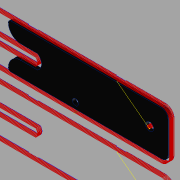
# Autodesk Inventor part: wheel_mount_brake
Saved by Autodesk Inventor 2021.3 (Build 253353000, 353)
## iProperties
Created: 2021-07-08
Part Number: wheel_mount_brake
Material: アルミニウム 6061
Document SubType Name: Modeling
Designer: gisen
Density: 2.7 g/cm^3
Appearance: アルミニウム - フラット
Author: gisen
Autodesk Inventor part; units mm, degrees
ref_plane "YZ Plane" through (0, 0, 0) normal (1, 0, 0) x (0, 1, 0)
ref_plane "XZ Plane" through (0, 0, 0) normal (0, 1, 0) x (-1, 0, 0)
ref_plane "XY Plane" through (0, 0, 0) normal (0, 0, 1) x (1, 0, 0)
ref_plane "作業平面1" through (0, 0, 0) normal (0, 0, 1) x (1, 0, 0)
sketch "スケッチ2" plane through (0, 0, 0) normal (0, 0, 1) x (1, 0, 0)
  line L0 (110, -57) -> (-20, -57)
  line L1 (-20, -57) -> (-20, -93)
  line L2 (-20, -93) -> (110, -93)
  line L3 (110, -93) -> (110, -57)
  circle A0 centre (0, -75) radius 6 construction
  circle A1 centre (0, -75) radius 75 construction
  point P0 (0, 0)
  dimension "d1" = 150
  dimension "d2" = 18
  dimension "d3" = 18
  dimension "d4" = 20
  dimension "d29" = 110
  constraints: 8 end point, 2 parallel, 1 horizontal, 1 perpendicular, 1 vertical alignment
  measures "d2" distance from line of L0 A0.centre
  measures "d3" distance from line of L2 A0.centre
  measures "d4" distance from line of L1 A0.centre
  measures "d29" distance from line of A0.centre L3
extrude "押し出し1" add sketch "スケッチ2" along normal blind 3
sketch "スケッチ3" plane through (0, 0, 3) normal (0, 0, 1) x (1, 0, 0)
  circle A0 centre (0, -75) radius 6 construction
  circle A1 centre (0, -75) radius 7
  line L0 (0, -68) -> (-38.1, -68) construction
  line L1 (-38.1, -68) -> (-38.1, -82) construction
  line L2 (-38.1, -82) -> (0, -82) construction
  line L3 (0, -82) -> (0, -68) construction
  line L4 (-20, -68) -> (-20, -82)
  line L5 (0, -82) -> (0, -68)
  line L6 (-20, -57) -> (-20, -93) projected
  line L7 (-20, -69.25) -> (3.9922, -69.25)
  line L8 (3.9922, -69.25) -> (3.9922, -80.75)
  line L9 (3.9922, -80.75) -> (-20, -80.75)
  line L10 (-20, -80.75) -> (-20, -69.25)
  point P0 (0, 0)
  point P1 (-3.9922, -80.75)
  point P2 (-3.9922, -69.25)
  point P3 (0, -80.75)
  point P4 (0, -69.25)
  point P5 (0, -82)
  dimension "d8" = 14
  dimension "d30" = 11.5
  constraints: 20 end point, 5 parallel, 3 point on circle, 2 horizontal, 2 perpendicular, 2 point on line, 2 tangent, 1 centre point, 1 coincident, 1 collinear
  measures "d8" diameter of A1
  measures "d30" distance between parallel lines of L7 L9
extrude "押し出し2" cut sketch "スケッチ3" against normal blind 14 contours A1 L8 | L8 L9 L5 L7 | L5 L9 A1 L7 | A1 L9 L4 L7
fillet "フィレット1" radius 10 2 edges at (-20, -80.75, 1.5) (-20, -69.25, 1.5)
ref_plane "作業平面2" through (-20, -75, 0) normal (0, -1, 0) x (1, 0, 0)
sketch "スケッチ4" plane through (0, 0, 3) normal (0, 0, 1) x (1, 0, 0)
  line L0 (-20, -93) -> (110, -93) projected
  line L1 (110, -57) -> (-20, -57) projected
  line L2 (110, -93) -> (110, -57) projected
  point P0 (0, 0)
  point P1 (95, -75)
  dimension "d25" = 15
  dimension "d26" = 36
  dimension "d27" = 18
  measures "d25" distance from line of L2 point (95, -75)
  measures "d26" distance between parallel lines of L0 L1
  measures "d27" distance from line of L1 point (95, -75)
hole "穴1" at (95, -75, 3) direction (0, 0, -1) diameter 6.6 end through all
fillet "フィレット2" radius 5 2 edges at (110, -57, 1.5) (110, -93, 1.5)
fillet "フィレット2" radius 2 2 edges at (-20, -57, 1.5) (-20, -93, 1.5)
ref_plane "作業平面3" through (0, -75, 0) normal (0, 0.7071068, 0.7071068) x (-1, 0, 0)
sketch "スケッチ5" plane through (0, 0, 3) normal (0, 0, 1) x (1, 0, 0)
  arc A0 (3.9922, -80.75) -> (3.9922, -69.25) centre (0, -75) ccw projected
  circle A1 centre (0, -75) radius 37 construction
  circle A2 centre (34.641, -88) radius 3.5 construction
  line L0 (-18, -93) -> (105, -93) construction
  point P0 (0, 0)
  dimension "d31" = 74
  dimension "d32" = 7
  dimension "d33" = 5
  constraints: 2 coincident, 1 centre point, 3 other
  measures "d32" diameter of A2
  measures "d33" distance from line of L0 A2.centre
hole "穴2" at (34.641, -88, 3) direction (0, 0, -1) diameter 5 end through all
equation "\"d3\" = d2"
equation "\"d9\" = d8"
equation "\"d27\" = 0.5 * d26"
